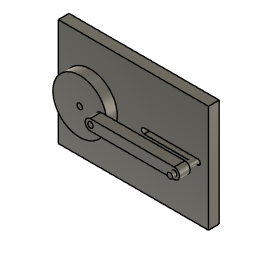
rotation to linear motion 1 v0 (Autodesk Fusion 360 design; units mm, degrees)
Autodesk Fusion 360 part; units mm, degrees
sketch "Sketch1" plane through (0, 0, 0) normal (0, 1, 0) x (1, 0, 0)
  line L0 (88.9, 63.5) -> (-88.9, 63.5)
  line L1 (-88.9, 63.5) -> (-88.9, -63.5)
  line L2 (-88.9, -63.5) -> (88.9, -63.5)
  line L3 (88.9, -63.5) -> (88.9, 63.5)
  line L4 (88.9, 63.5) -> (-88.9, -63.5) construction
  line L5 (-88.9, 63.5) -> (88.9, -63.5) construction
  constraint horizontal L0
  constraint perpendicular L0 L1
  constraint parallel L0 L2
  constraint parallel L1 L3
  constraint coincident L4 origin
  constraint coincident L5 origin
extrude "Extrude1" add sketch "Sketch1" along normal blind 12.7 makes body 1 in component "Base"
sketch "Sketch2" plane through (0, 0, 0) normal (0, -1, 0) x (1, 0, 0)
  line L0 (88.9, -63.5) -> (88.9, 63.5)
  line L1 (88.9, 63.5) -> (-88.9, 63.5)
  line L2 (-88.9, 63.5) -> (-88.9, -63.5)
  line L3 (-88.9, -63.5) -> (88.9, -63.5)
  circle A0 centre (-50.8, 0) radius 3.175
  dimension "d3" = 6.35
  measures "d3" diameter of A0
extrude "Extrude2" add sketch "Sketch2" along normal blind 12.7 contours A0 bodies 1 in component "Base"
sketch "Sketch3" plane through (0, 0, 0) normal (0, -1, 0) x (1, 0, 0)
  circle A0 centre (-50.8, 0) radius 3.175
  line L0 (88.9, -63.5) -> (88.9, 63.5)
  line L1 (88.9, 63.5) -> (-88.9, 63.5)
  line L2 (-88.9, 63.5) -> (-88.9, -63.5)
  line L3 (-88.9, -63.5) -> (88.9, -63.5)
  circle A1 centre (-50.8, 0) radius 31.75
  dimension "d6" = 63.5
  constraint concentric A0 A1
  measures "d6" diameter of A1
extrude "Extrude1'" add sketch "Sketch3" along normal blind 12.7 separate body contours A1 makes body 2 in component "Wheel"
sketch "Sketch4" plane through (0, -12.7, 0) normal (0, -1, 0) x (1, 0, 0)
  circle A0 centre (-50.8, 0) radius 3.175
  circle A1 centre (-50.8, 0) radius 31.75
  circle A2 centre (-25.4, 0) radius 3.175
  dimension "d9" = 6.35
  measures "d9" diameter of A2
extrude "Extrude2'" add sketch "Sketch4" along normal blind 12.7 contours A2 bodies 2 in component "Wheel"
sketch "Sketch5" plane through (0, 0, 0) normal (0, -1, 0) x (1, 0, 0)
  circle A0 centre (-50.8, 0) radius 3.175
  line L0 (88.9, -63.5) -> (88.9, 63.5)
  line L1 (88.9, 63.5) -> (-88.9, 63.5)
  line L2 (-88.9, 63.5) -> (-88.9, -63.5)
  line L3 (-88.9, -63.5) -> (88.9, -63.5)
  line L4 (12.7, -3.175) -> (76.2, -3.175)
  arc A1 (76.2, -3.175) -> (76.2, 3.175) centre (76.2, 0) ccw
  line L5 (76.2, 3.175) -> (12.7, 3.175)
  arc A2 (12.7, 3.175) -> (12.7, -3.175) centre (12.7, 0) ccw
  line L6 (12.7, 0) -> (76.2, 0) construction
  dimension "d12" = 6.35
  constraint tangent L4 A1
  constraint tangent A1 L5
  constraint parallel L4 L5
  constraint tangent L5 A2
  constraint tangent L4 A2
  constraint horizontal L6
  measures "d12" diameter of A1
extrude "Extrude3" cut sketch "Sketch5" against normal blind 12.7 contours L4 A1 L5 A2 bodies 1 in component "Base"
sketch "Sketch6" plane through (0, -25.4, 0) normal (0, -1, 0) x (1, 0, 0)
  circle A0 centre (-25.4, 0) radius 3.175
  circle A1 centre (73.66, 0) radius 3.175
  dimension "d15" = 6.35
  measures "d15" diameter of A1
extrude "Extrude1''" add sketch "Sketch6" along normal blind -43.18 and the other way blind -5.08 separate body contours A1 makes body 3 in component "Slide"
sketch "Sketch7" plane through (0, -25.4, 0) normal (0, -1, 0) x (1, 0, 0)
  circle A0 centre (-25.4, 0) radius 3.175
  circle A1 centre (-25.4, 0) radius 3.175
  circle A2 centre (73.66, 0) radius 3.175
  circle A3 centre (-25.4, 0) radius 6.35
  circle A4 centre (73.66, 0) radius 6.35
  line L0 (-25.6943, 6.3432) -> (73.6596, 6.35)
  line L1 (-25.6943, -6.3432) -> (73.6596, -6.35)
  dimension "d20" = 12.7
  dimension "d21" = 12.7
  constraint concentric A1 A3
  constraint concentric A2 A4
  constraint coincident A3 L0.start
  constraint coincident A4 L0.end
  constraint tangent A4 L0
  constraint coincident A3 L1.start
  constraint coincident A4 L1.end
  constraint tangent A4 L1
  measures "d20" diameter of A3
  measures "d21" diameter of A4
extrude "Extrude1'''" add sketch "Sketch7" against normal blind 12.7 separate body contours A3 L0 L1 | A3 A4 L0 L1 | A4 makes body 4 in component "Component"
component "Base" placed x (1, 0, 0) y (0, 1, 0) z (0, 0, 1) at (0, 0, 0)
component "Wheel" placed x (1, 0, 0) y (0, 1, 0) z (0, 0, 1) at (0, 0, 0)
component "Slide" placed x (1, 0, 0) y (0, 1, 0) z (0, 0, 1) at (0, 0, 0)
component "Component" placed x (1, 0, 0) y (0, 1, 0) z (0, 0, 1) at (0, 0, 0)
